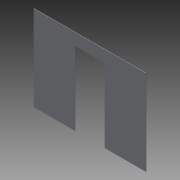
# Autodesk Inventor part: Wall_door
Saved by Autodesk Inventor 2013 (Build 170138000, 138)
## iProperties
Created: 2011-06-21
Part Number: Wall_door
Document SubType Name: Modeling
Designer: rrw
Density: 1 g/cm^3
Material: Generic
Author: rrw
Autodesk Inventor part; units mm, degrees
ref_plane "YZ Plane" through (0, 0, 0) normal (1, 0, 0) x (0, 1, 0)
ref_plane "XZ Plane" through (0, 0, 0) normal (0, 1, 0) x (-1, 0, 0)
ref_plane "XY Plane" through (0, 0, 0) normal (0, 0, 1) x (1, 0, 0)
sketch "Sketch1" plane through (0, 0, 0) normal (0, 0, 1) x (1, 0, 0)
  line L0 (-840.6501, 1205.233) -> (1959.3499, 1205.233)
  line L1 (1959.3499, 1205.233) -> (1959.3499, -924.767)
  line L2 (1959.3499, -924.767) -> (-840.6501, -924.767)
  line L3 (-840.6501, -924.767) -> (-840.6501, 1205.233)
  line L4 (189.3499, -924.767) -> (929.3499, -924.767)
  line L5 (929.3499, -924.767) -> (929.3499, 905.233)
  line L6 (929.3499, 905.233) -> (189.3499, 905.233)
  line L7 (189.3499, 905.233) -> (189.3499, -924.767)
  point P0 (0, 0)
  dimension "d0" = 2800
  dimension "d1" = 2130
  dimension "d3" = 740
  dimension "d4" = 1830
  dimension "d5" = 1030
  constraints: 16 end point, 4 parallel, 2 horizontal, 2 perpendicular, 1 point on line
  measures "d0" distance of L1.end L2.end
  measures "d1" distance of L0.end L1.end
  measures "d3" distance of L6.end L5.end
  measures "d4" distance of L5.end L4.end
  measures "d5" distance between parallel lines of L7 L3
extrude "Extrusion1" add sketch "Sketch1" along normal blind 10 contours L0 L1 L2 L5 L6 L7 L3
body "Solid1"
